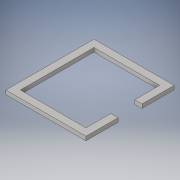
# Autodesk Inventor part: Front_chasis
Saved by Autodesk Inventor 2016 (Build 200138000, 138)
## iProperties
Created: 2016-02-28
Part Number: Front_chasis
Material: Generic
Document SubType Name: Modeling
Designer: torti_000
Density: 1 g/cm^3
Appearance: Default
Author: torti_000
Autodesk Inventor part; units mm, degrees
ref_plane "YZ Plane" through (0, 0, 0) normal (1, 0, 0) x (0, 1, 0)
ref_plane "XZ Plane" through (0, 0, 0) normal (0, 1, 0) x (-1, 0, 0)
ref_plane "XY Plane" through (0, 0, 0) normal (0, 0, 1) x (1, 0, 0)
sketch "Sketch1" plane through (0, 0, 0) normal (0, 1, 0) x (-1, 0, 0)
  line L0 (0, -57.15) -> (11.43, -57.15)
  line L1 (11.43, -95.25) -> (0, -95.25)
  line L2 (0, -57.15) -> (0, -6.35)
  line L3 (0, -95.25) -> (0, -146.05)
  line L4 (0, -146.05) -> (127, -146.05)
  line L5 (127, -146.05) -> (127, -6.35)
  line L6 (127, -6.35) -> (0, -6.35)
  line L7 (11.43, -17.78) -> (11.43, -45.72)
  line L8 (11.43, -106.68) -> (11.43, -134.62)
  line L9 (11.43, -134.62) -> (115.57, -134.62)
  line L10 (115.57, -134.62) -> (115.57, -17.78)
  line L11 (115.57, -17.78) -> (11.43, -17.78)
  line L12 (11.43, -45.72) -> (11.43, -57.15)
  line L13 (11.43, -106.68) -> (11.43, -95.25)
  point P0 (0, 0)
  dimension "d4" = 50.8
  dimension "d5" = 50.8
  dimension "d6" = 127
  dimension "d7" = 11.43
  constraints: 28 end point, 6 perpendicular, 2 vertical, 1 point on line, 3 other
  measures "d4" distance of L0.start L2.end
  measures "d5" distance of L1.end L3.end
  measures "d6" distance of L3.end L4.end
  measures "d7" distance between parallel lines of L6 L11
extrude "Extrusion1" add sketch "Sketch1" along normal blind 6.35
body "Solid1"
